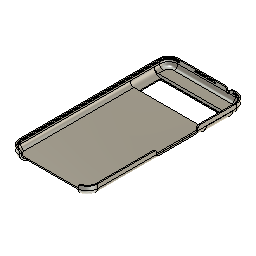
Phone Case (Autodesk Fusion 360 design; units mm, degrees)
Autodesk Fusion 360 part; units mm, degrees
note: some values were not read from the file. Chosen so that the rebuilt part matches the saved one: which bodies a step acts on; which sketch regions a step uses; a direction; which face or edge a step refers to.
sketch "Base Profile" plane through (0, 0, 0) normal (0, 1, 0) x (1, 0, 0)
  line L0 (-39.6, 0) -> (39.6, 0) construction
  line L1 (0, 8.3) -> (-35.6374, 8.3)
  arc A0 (-35.6374, 8.3) -> (-39.6372, 4.2651) centre (-35.6374, 4.3) ccw
  line L2 (0, 9.6) -> (-35.6374, 9.6)
  arc A1 (-35.6374, 9.6) -> (-40.9346, 4.1273) centre (-35.6374, 4.3) ccw
  line L3 (-40.9346, 4.1273) -> (-40.8, 0)
  line L4 (0, 0) -> (0, 9.6)
  line L5 (-39.6372, 4.2651) -> (-39.6, 0)
  line L6 (-40.8, 0) -> (-39.6, 0)
  point P0 (-39.6, 8.3)
  dimension "d2" = 8.3
  dimension "d3" = 4
  dimension "d37" = 90.5
  dimension "d38" = 1.2
  dimension "d39" = 39.6
  dimension "d40" = 4.3
  constraint horizontal L0
  constraint horizontal L1
  constraint coincident P0 L1
  constraint tangent L1 A0
  constraint midpoint L4.start L0
  constraint coincident L4.start origin
  constraint perpendicular L2 L4
  constraint parallel L0 L6
  constraint concentric A0 A1
  constraint tangent L2 A1
  constraint coincident L4 L1.start
  constraint tangent A0 L5
  constraint tangent A1 L3
  measures "d2" distance of L0.start P0
  measures "d3" radius of A0
  measures "d37" angle of L0 L5
  measures "d38" distance of L0.start L3.end
  measures "d39" distance of L4.start L0.start
  measures "d40" distance of L0 A0.centre
sketch "Perimeter" plane through (0, 0, 0) normal (0, 0, 1) x (1, 0, 0)
  line L0 (-30.1, 82.05) -> (30.1, 82.05)
  line L1 (39.6, 72.55) -> (39.6, -72.55)
  line L2 (30.1, -82.05) -> (-30.1, -82.05)
  line L3 (-39.6, -72.55) -> (-39.6, 72.55)
  line L4 (-39.6, 82.05) -> (39.6, -82.05) construction
  line L5 (39.6, 82.05) -> (-39.6, -82.05) construction
  arc A0 (-30.1, 82.05) -> (-39.6, 72.55) centre (-30.1, 72.55) ccw
  line L6 (-30.1, 72.55) -> (30.1, 72.55) construction
  line L7 (30.1, 72.55) -> (30.1, -72.55) construction
  line L8 (30.1, -72.55) -> (-30.1, -72.55) construction
  line L9 (-30.1, -72.55) -> (-30.1, 72.55) construction
  line L10 (30.1, -72.55) -> (-30.1, 72.55) construction
  arc A1 (-39.6, -72.55) -> (-30.1, -82.05) centre (-30.1, -72.55) ccw
  arc A2 (30.1, -82.05) -> (39.6, -72.55) centre (30.1, -72.55) ccw
  arc A3 (39.6, 72.55) -> (30.1, 82.05) centre (30.1, 72.55) ccw
  line L11 (-39.6, -82.05) -> (-39.6, -72.55) construction
  line L12 (-30.1, -82.05) -> (-39.6, -82.05) construction
  line L13 (39.6, -82.05) -> (30.1, -82.05) construction
  line L14 (39.6, -72.55) -> (39.6, -82.05) construction
  line L15 (30.1, 82.05) -> (39.6, 82.05) construction
  line L16 (39.6, 82.05) -> (39.6, 72.55) construction
  line L17 (-39.6, 72.55) -> (-39.6, 82.05) construction
  line L18 (-39.6, 82.05) -> (-30.1, 82.05) construction
  point P0 (39.6, 0)
  dimension "d9" = 164.1
  dimension "d10" = 9.5
  constraint horizontal L0
  constraint perpendicular L0 L1
  constraint parallel L0 L2
  constraint parallel L1 L3
  constraint coincident L4 origin
  constraint coincident L5 origin
  constraint coincident L1 P0
  constraint tangent L3 A0
  constraint tangent L0 A0
  constraint horizontal L6
  constraint vertical L7
  constraint horizontal L8
  constraint vertical L9
  constraint coincident A0.centre L6.start
  constraint midpoint origin L10
  constraint coincident L8.end L9.start
  constraint coincident L7.end L8.start
  constraint coincident L6.end L7.start
  constraint equal A0 A1
  constraint equal A0 A2
  constraint equal A0 A3
  constraint parallel L1 L11
  constraint parallel L0 L12
  constraint parallel L0 L13
  constraint perpendicular L0 L14
  constraint horizontal L15
  constraint perpendicular L0 L16
  constraint parallel L1 L17
  constraint horizontal L18
  measures "d9" distance of L4.start L5.end
  measures "d10" radius of A0
sweep "Sweep1" add profiles "Base Profile" path "Perimeter" along A0 L0 A3 L1 A2 L2 A1 L3 section 1 makes body 1
sketch "Headphone notch" plane through (0, 82.0438, 0.716) normal (0, -0.999962, -0.008727) x (1, 0, 0)
  line L0 (-30.1, 0) -> (-30.1, -4.3)
  arc A0 (21.1007, -4.2633) -> (24.0993, -4.2633) centre (22.6, -4.216) ccw
  line L1 (22.6, -4.216) -> (22.6, 0) construction
  line L2 (-30.1, -0.716) -> (-30.1, -4.9813)
  line L3 (-30.1, -4.9813) -> (30.1, -4.9813)
  line L4 (30.1, -4.9813) -> (30.1, -0.716)
  line L5 (30.1, -0.716) -> (-30.1, -0.716)
  arc A1 (21.05, -2.653) -> (19.051, -0.716) centre (19.051, -2.716) ccw
  line L6 (-30.1, -0.716) -> (30.1, -0.716)
  line L7 (21.1007, -4.2633) -> (21.05, -2.653)
  arc A2 (26.149, -0.716) -> (24.15, -2.653) centre (26.149, -2.716) ccw
  line L8 (24.0993, -4.2633) -> (24.15, -2.653)
  point P0 (39.6372, -4.2651)
  dimension "d17" = 3
  dimension "d43" = 22.6
  dimension "d44" = 2
  dimension "d45" = 3.5
  dimension "d46" = 3.1
  constraint coincident A0.centre L1.start
  constraint coincident L5 A1.end
  constraint tangent L5 A1
  constraint vertical L1
  constraint horizontal A0.start A0.end
  constraint tangent A0 L7
  constraint tangent A1 L7
  constraint symmetric A0.start L1 A0.end
  constraint symmetric L1 A1.start A2.end
  constraint symmetric L1 A1.end A2.start
  constraint symmetric L1 A1 A2
  measures "d17" diameter of A0
  measures "d43" distance of origin L1
  measures "d44" radius of A1
  measures "d45" distance of A0.centre L6
  measures "d46" distance of A1.start A2.end
extrude "Extrude2" cut sketch "Headphone notch" along normal mid plane 10 contours A0 L3 L5 A1 L6 L7 A2 L8 | A0 L3 bodies 1
sketch "Volume control notch" plane through (39.597, 0, 0.3456) normal (-0.999962, 0, -0.008727) x (0, -1, 0)
  line L0 (-28.6516, -7.3456) -> (7.6516, -7.3456)
  line L1 (-10.5, -7.3456) -> (-10.5, -0.3456) construction
  arc A0 (-32.15, -3.9506) -> (-28.6516, -7.3456) centre (-28.6516, -3.8456) ccw
  line L2 (-32.15, -3.9506) -> (-32.2, -2.2855)
  arc A1 (-32.2, -2.2855) -> (-34.1991, -0.3456) centre (-34.1991, -2.3456) ccw
  arc A2 (7.6516, -7.3456) -> (11.15, -3.9506) centre (7.6516, -3.8456) ccw
  line L3 (11.15, -3.9506) -> (11.2, -2.2855)
  arc A3 (13.1991, -0.3456) -> (11.2, -2.2855) centre (13.1991, -2.3456) ccw
  line L4 (-72.55, -0.3456) -> (-72.55, -4.6108)
  line L5 (-72.55, -4.6108) -> (72.55, -4.6108)
  line L6 (72.55, -4.6108) -> (72.55, -0.3456)
  line L7 (72.55, -0.3456) -> (-72.55, -0.3456)
  dimension "d25" = 7
  dimension "d26" = 2
  dimension "d27" = 3.5
  dimension "d29" = 43.4
  dimension "d30" = 43.3
  dimension "d47" = 10.5
  constraint coincident L0 L1.start
  constraint midpoint L0 L1.start
  constraint tangent L0 A0
  constraint tangent A0 L2
  constraint tangent L2 A1
  constraint symmetric L0.start L1 L0.end
  constraint symmetric L1 A0.start A2.end
  constraint symmetric L1 A0 A2
  constraint symmetric L1 L2.end L3.end
  constraint symmetric L1 A1.end A3.start
  constraint symmetric L1 A1 A3
  constraint coincident A1.end L7
  constraint tangent A1 L7
  constraint horizontal L0
  constraint vertical L1
  constraint coincident L1.end L7
  measures "d25" distance of L1.start L1.end
  measures "d26" radius of A1
  measures "d27" radius of A0
  measures "d29" distance of L2.end L3.end
  measures "d30" distance of A0.start A2.end
  measures "d47" distance of origin L1
extrude "Extrude3" cut sketch "Volume control notch" along normal mid plane 10 contours L0 A0 A2 L5 | A0 L2 A1 A2 L3 A3 L5 L7 bodies 1
sketch "Charger notch" plane through (0, 0, -9.6) normal (0, 0, -1) x (1, 0, 0)
  arc A0 (-35.6374, -72.55) -> (-30.1, -78.0874) centre (-30.1, -72.55) ccw
  line L0 (-30.1, -78.0874) -> (30.1, -78.0874)
  arc A1 (30.1, -78.0874) -> (35.6374, -72.55) centre (30.1, -72.55) ccw
  line L1 (35.6374, -72.55) -> (35.6374, 72.55)
  arc A2 (35.6374, 72.55) -> (30.1, 78.0874) centre (30.1, 72.55) ccw
  line L2 (30.1, 78.0874) -> (-30.1, 78.0874)
  arc A3 (-30.1, 78.0874) -> (-35.6374, 72.55) centre (-30.1, 72.55) ccw
  line L3 (-35.6374, 72.55) -> (-35.6374, -72.55)
  line L4 (30.1, 82.05) -> (-30.1, 82.05) construction
  line L5 (30.1, 83.25) -> (-30.1, 83.25) construction
  line L6 (30.1, 83.3846) -> (-30.1, 83.3846)
  line L7 (-25.2845, 77.9846) -> (27.2845, 77.9846)
  line L8 (-29.6, 83.3846) -> (31.6, 83.3846)
  line L9 (1, 83.3846) -> (1, 77.9846) construction
  arc A4 (-27.0092, 78.9719) -> (-25.2845, 77.9846) centre (-25.2845, 79.9846) ccw
  line L10 (-27.0092, 78.9719) -> (-29.6, 83.3846)
  line L11 (29.0092, 78.9719) -> (31.6, 83.3846)
  arc A5 (27.2845, 77.9846) -> (29.0092, 78.9719) centre (27.2845, 79.9846) ccw
  line L12 (31.6, 83.3846) -> (31.6, 86.3846)
  line L13 (-29.6, 83.3846) -> (-29.6, 86.3846)
  line L14 (-29.6, 86.3846) -> (31.6, 86.3846)
  dimension "d48" = 52.569
  dimension "d49" = 61.2
  dimension "d50" = 2
  dimension "d51" = 5.4
  dimension "d52" = 1
  dimension "d55" = 3
  constraint parallel L4 L7
  constraint horizontal L8
  constraint midpoint L8 L9.start
  constraint midpoint L7 L9.end
  constraint vertical L9
  constraint tangent L7 A4
  constraint tangent A4 L10
  constraint collinear L6 L8
  constraint symmetric L7.start L9 L7.end
  constraint symmetric L8.start L9 L8.end
  constraint symmetric L9 A4.start L11.start
  constraint symmetric L9 A4 A5
  constraint perpendicular L8 L12
  constraint perpendicular L8 L13
  constraint horizontal L14
  measures "d48" distance of L7.start L7.end
  measures "d49" distance of L8.start L8.end
  measures "d50" radius of A4
  measures "d51" distance of L7 L8
  measures "d52" distance of origin L9
  measures "d55" distance of L8.end L12.end
extrude "Extrude4" cut sketch "Charger notch" against normal blind 11.927 contours L2 L6 L8 A4 L10 L11 A5 | L6 L8 L12 L13 L14 bodies 1
fillet "Fillet2" radius 2 2 edges at (31.1353, -82.5931, 0) (-29.1687, -82.65, 0) on bodies 1
sketch "Retaining Ring profile for sweep" plane through (0, 0, 0) normal (0, 1, 0) x (1, 0, 0)
  line L0 (-39.6372, 4.2651) -> (-39.6, 0)
  line L1 (-39.6175, 2) -> (-38.6087, 1.4293)
  line L2 (-38.6087, 1.4293) -> (-38.6087, 1.0087)
  line L3 (-38.6087, 1.0087) -> (-39.6087, 1)
  dimension "d60" = 60
  dimension "d62" = 1
  dimension "d63" = 1
  dimension "d64" = 1
  constraint coincident L0 L1.start
  constraint vertical L2
  constraint coincident L0 L3.end
  constraint perpendicular L0 L3
  measures "d60" angle of L0 L1
  measures "d62" vertical distance of L1.start L3.end
  measures "d63" vertical distance of L0.end L3.end
  measures "d64" horizontal distance of L2.end L3.end
sweep "Sweep2" add profiles "Retaining Ring profile for sweep" path "Perimeter" along A0 L0 A3 L1 A2 L2 A1 L3 section 1 separate body makes body 2
sketch "Retaining Ring cutouts" plane through (0, 0, 0) normal (0, 0, 1) x (1, 0, 0)
  line L0 (-28.3042, 76.8842) -> (-11.4621, 76.8842)
  line L1 (-11.4621, 76.8842) -> (-11.4621, 87.5508)
  line L2 (-11.4621, 87.5508) -> (-28.3042, 87.5508)
  line L3 (-28.3042, 87.5508) -> (-28.3042, 76.8842)
  line L4 (9.7778, 73.0492) -> (28.2586, 73.0492)
  line L5 (28.2586, 73.0492) -> (28.2586, 87.5508)
  line L6 (28.2586, 87.5508) -> (9.7778, 87.5508)
  line L7 (9.7778, 87.5508) -> (9.7778, 73.0492)
  line L8 (34.3544, -16.9326) -> (47.9088, -16.9326)
  line L9 (47.9088, -16.9326) -> (47.9088, 41.7139)
  line L10 (47.9088, 41.7139) -> (34.3544, 41.7139)
  line L11 (34.3544, 41.7139) -> (34.3544, -16.9326)
  line L12 (-32.3646, -87.8519) -> (33.749, -87.8519)
  line L13 (33.749, -87.8519) -> (33.749, -78.2722)
  line L14 (33.749, -78.2722) -> (-32.3646, -78.2722)
  line L15 (-32.3646, -78.2722) -> (-32.3646, -87.8519)
  constraint horizontal L0
  constraint vertical L1
  constraint horizontal L2
  constraint vertical L3
  constraint horizontal L4
  constraint vertical L5
  constraint horizontal L6
  constraint vertical L7
  constraint horizontal L8
  constraint vertical L9
  constraint horizontal L10
  constraint vertical L11
  constraint horizontal L12
  constraint vertical L13
  constraint horizontal L14
  constraint vertical L15
extrude "Extrude5" cut sketch "Retaining Ring cutouts" against normal blind 10 bodies 2 makes body 3 at (-4.3822, 81.395, -1.6195) makes body 4 at (38.945, 62.2713, -1.6195) makes body 5 at (-38.945, 24.1833, -1.6195)
combine "Combine1" operation add target body 1 tool bodies 2 3 4 5
ref_plane "WorkPlane1" through (0, 40.9, 0) normal (0, 1, 0) x (0, 0, 1)
sketch "Camera Hump" plane through (0, 40.9, 0) normal (0, 1, 0) x (1, 0, 0)
  line L0 (-30.1, 9.6) -> (-35.6374, 9.6)
  line L1 (-30.1, 9.6) -> (30.1, 9.6)
  line L2 (35.6374, 9.6) -> (30.1, 9.6)
  line L3 (35.6374, 9.6) -> (30.1, 9.6)
  line L4 (30.1, 9.6) -> (27.9175, 9.6)
  line L5 (27.9175, 9.6) -> (-25.9175, 9.6)
  line L6 (-25.9175, 9.6) -> (-30.1, 9.6)
  line L7 (-30.1, 9.6) -> (-35.6374, 9.6)
  spline S0 degree 3 poles (40.201, 6.995) (40.201, 6.995) (40.2595, 6.9015) (40.4476, 6.5348) (40.5721, 6.2617) (40.7754, 5.6397) (40.8693, 5.25) (40.9338, 4.5974) (40.9422, 4.3628) (40.9346, 4.1273) knots 0 0 0 0 0.136028 0.136028 0.272056 0.272056 0.404552 0.404552 0.473854 0.473854 0.473854 0.473854
  arc A0 (40.9346, 4.1273) -> (35.6374, 9.6) centre (35.6374, 4.3) ccw
  arc A1 (40.9346, 4.1273) -> (35.6374, 9.6) centre (35.6374, 4.3) ccw
  spline S1 degree 3 poles (40.9346, 4.1273) (40.9422, 4.3628) (40.9338, 4.5974) (40.8693, 5.25) (40.7754, 5.6397) (40.5721, 6.2617) (40.4476, 6.5348) (40.2595, 6.9015) (40.201, 6.995) (40.201, 6.995) knots -0.473854 -0.473854 -0.473854 -0.473854 -0.404552 -0.404552 -0.272056 -0.272056 -0.136028 -0.136028 0 0 0 0
  arc A2 (-35.6374, 9.6) -> (-40.9346, 4.1273) centre (-35.6374, 4.3) ccw
  arc A3 (-35.6374, 9.6) -> (-40.9346, 4.1273) centre (-35.6374, 4.3) ccw
  line L8 (-30.1, 8.3) -> (-35.6374, 8.3)
  line L9 (-30.1, 8.3) -> (-25.9175, 8.3)
  line L10 (-25.9175, 8.3) -> (27.9175, 8.3)
  line L11 (27.9175, 8.3) -> (30.1, 8.3)
  line L12 (35.6374, 8.3) -> (30.1, 8.3)
  line L13 (35.6374, 8.3) -> (30.1, 8.3)
  line L14 (30.1, 8.3) -> (-30.1, 8.3)
  line L15 (-30.1, 8.3) -> (-35.6374, 8.3)
  arc A4 (-35.6374, 8.3) -> (-39.6372, 4.2651) centre (-35.6374, 4.3) ccw
  arc A5 (-35.6374, 8.3) -> (-39.6372, 4.2651) centre (-35.6374, 4.3) ccw
  spline S2 degree 3 poles (39.6372, 4.2651) (39.6404, 4.6245) (39.5922, 4.9872) (39.4158, 5.6618) (39.283, 5.968) (39.024, 6.4461) (38.8756, 6.655) (38.6508, 6.9366) (38.5803, 7.0091) (38.5802, 7.0092) knots 0.67617 0.67617 0.67617 0.67617 0.785853 0.785853 0.904084 0.904084 1.023831 1.023831 1.143577 1.143577 1.143577 1.143577
  spline S3 degree 3 poles (38.5802, 7.0092) (38.5803, 7.0091) (38.6508, 6.9366) (38.8756, 6.655) (39.024, 6.4461) (39.283, 5.968) (39.4158, 5.6618) (39.5922, 4.9872) (39.6404, 4.6245) (39.6372, 4.2651) knots 1.143577 1.143577 1.143577 1.143577 1.263323 1.263323 1.38307 1.38307 1.501301 1.501301 1.610984 1.610984 1.610984 1.610984
  arc A6 (39.6372, 4.2651) -> (35.6374, 8.3) centre (35.6374, 4.3) ccw
  arc A7 (39.6372, 4.2651) -> (35.6374, 8.3) centre (35.6374, 4.3) ccw
  line L16 (0, 8.3) -> (0, 12.3) construction
  line L17 (-32.9364, 12.3) -> (32.9364, 12.3)
  arc A8 (-32.9364, 12.3) -> (-40.9346, 4.1273) centre (-32.9364, 4.3) ccw
  arc A9 (40.9346, 4.1273) -> (32.9364, 12.3) centre (32.9364, 4.3) ccw
  dimension "d79" = 4
  constraint midpoint L14 L16.start
  constraint perpendicular L5 L16
  constraint horizontal L17
  constraint midpoint L16.end L17
  constraint coincident A2 A3.end
  constraint tangent L17 A8
  constraint coincident A2.end A3.end
  constraint horizontal A2.centre A8.centre
  constraint symmetric L16 L17.start L17.end
  constraint symmetric L16 A2.end S0.end
  constraint symmetric L16 A8 A9
  measures "d79" distance of L16.start L16.end
extrude "Extrude7" add sketch "Camera Hump" along normal blind 27.3 bodies 1
sketch "Camera Hump Hole" plane through (0, 0, -12.3) normal (0, 0, -1) x (1, 0, 0)
  line L0 (32.9364, -40.9) -> (-32.9364, -40.9)
  line L1 (-32.9364, -40.9) -> (-32.9364, -68.2)
  line L2 (-32.9364, -68.2) -> (32.9364, -68.2)
  line L3 (32.9364, -68.2) -> (32.9364, -40.9)
  line L4 (36.25, -66.7) -> (-34.25, -66.7)
  line L5 (-34.25, -66.7) -> (-34.25, -42.4)
  line L6 (-34.25, -42.4) -> (36.25, -42.4)
  line L7 (36.25, -42.4) -> (36.25, -66.7)
  line L8 (-34.25, -54.55) -> (-32.9364, -54.55) construction
  point P0 (1, -42.4)
  dimension "d82" = 1
  dimension "d83" = 24.3
  dimension "d84" = 70.5
  constraint horizontal L4
  constraint vertical L5
  constraint horizontal L6
  constraint vertical L7
  constraint midpoint L5 L8.start
  constraint midpoint L1 L8.end
  constraint horizontal L8
  constraint midpoint L6 P0
  measures "d82" horizontal distance of origin P0
  measures "d83" distance of L4.start L6.end
  measures "d84" distance of L5.end L6.end
extrude "Extrude8" cut sketch "Camera Hump Hole" against normal through all contours L1 L3 L4 L6 bodies 1
fillet "Fillet3" radius 3 4 edges at (32.9364, 66.7, -10.3) (32.9364, 42.4, -10.3) (-32.9364, 42.4, -10.3) (-32.9364, 66.7, -10.3) on bodies 1
ref_plane "WorkPlane2" through (0, 54.55, -10.3) normal (0, -1, 0) x (1, 0, 0)
sketch "Camera Hump Internal Cutout" plane through (0, 54.55, 0) normal (0, -1, 0) x (1, 0, 0)
  line L0 (-29.9364, -8.3) -> (-29.9364, -12.3) construction
  line L1 (-29.9364, -12.3) -> (29.9364, -12.3)
  line L2 (29.9364, -12.3) -> (29.9364, -8.3) construction
  line L3 (29.9364, -8.3) -> (-29.9364, -8.3)
  line L4 (-29.9364, -8.3) -> (29.9364, -8.3)
  line L5 (32.9364, -8.3) -> (29.9364, -8.3)
  line L6 (32.9364, -8.3) -> (29.9364, -8.3)
  line L7 (29.9364, -8.3) -> (-29.9364, -8.3)
  line L8 (-29.9364, -8.3) -> (-32.9364, -8.3)
  line L9 (-29.9364, -8.3) -> (-32.9364, -8.3)
  line L10 (-35.6374, -8.3) -> (-30.1, -8.3)
  line L11 (-30.1, -8.3) -> (-25.9175, -8.3)
  line L12 (-25.9175, -8.3) -> (27.9175, -8.3)
  line L13 (27.9175, -8.3) -> (30.1, -8.3)
  line L14 (30.1, -8.3) -> (35.6374, -8.3)
  line L15 (30.1, -8.3) -> (35.6374, -8.3)
  line L16 (30.1, -8.3) -> (-30.1, -8.3)
  line L17 (-35.6374, -8.3) -> (-30.1, -8.3)
  arc A0 (32.9364, -12.3) -> (40.9346, -4.4727) centre (32.9364, -4.3) ccw
  arc A1 (32.9364, -12.3) -> (40.9346, -4.4727) centre (32.9364, -4.3) ccw
  arc A2 (-40.9346, -4.4727) -> (-32.9364, -12.3) centre (-32.9364, -4.3) ccw
  arc A3 (-40.9346, -4.4727) -> (-32.9364, -12.3) centre (-32.9364, -4.3) ccw
  line L18 (29.9364, -12.3) -> (-29.9364, -12.3)
  line L19 (32.9364, -12.3) -> (32.9364, -8.3)
  line L20 (32.9364, -8.3) -> (32.9364, -12.3) construction
  arc A4 (-39.6372, -4.2651) -> (-35.6374, -8.3) centre (-35.6374, -4.3) ccw
  arc A5 (-39.6372, -4.2651) -> (-35.6374, -8.3) centre (-35.6374, -4.3) ccw
  spline S0 degree 3 poles (39.6372, -4.2651) (39.6404, -4.6245) (39.5922, -4.9872) (39.4158, -5.6618) (39.283, -5.968) (39.024, -6.4461) (38.8756, -6.655) (38.6508, -6.9366) (38.5803, -7.0091) (38.5802, -7.0092) knots 0.67617 0.67617 0.67617 0.67617 0.785853 0.785853 0.904084 0.904084 1.023831 1.023831 1.143577 1.143577 1.143577 1.143577
  spline S1 degree 3 poles (38.5802, -7.0092) (38.5803, -7.0091) (38.6508, -6.9366) (38.8756, -6.655) (39.024, -6.4461) (39.283, -5.968) (39.4158, -5.6618) (39.5922, -4.9872) (39.6404, -4.6245) (39.6372, -4.2651) knots 1.143577 1.143577 1.143577 1.143577 1.263323 1.263323 1.38307 1.38307 1.501301 1.501301 1.610984 1.610984 1.610984 1.610984
  arc A6 (35.6374, -8.3) -> (39.6372, -4.2651) centre (35.6374, -4.3) ccw
  arc A7 (35.6374, -8.3) -> (39.6372, -4.2651) centre (35.6374, -4.3) ccw
  line L21 (32.9364, -11.3) -> (-32.9364, -11.3)
  line L22 (0, 0) -> (0, -11.3) construction
  arc A8 (-39.6372, -4.2651) -> (-32.9364, -11.3) centre (-32.9364, -4.5913) ccw
  arc A9 (32.9364, -11.3) -> (39.6372, -4.2651) centre (32.9364, -4.5913) ccw
  dimension "d89" = 1
  constraint horizontal L21
  constraint coincident L22.start origin
  constraint perpendicular L12 L22
  constraint midpoint L21 L22.end
  constraint coincident A4.start A5.start
  constraint tangent L21 A8
  constraint vertical A2.centre A8.centre
  constraint symmetric L21.end L22 L21.start
  constraint symmetric L22 A4.start S0.start
  constraint symmetric L22 A8 A9
  measures "d89" distance of L1 L21
extrude "Extrude9" cut sketch "Camera Hump Internal Cutout" along normal mid plane 25.2 bodies 1
equation "d9 = 40.4 mm + 148.3 mm - 24.6 mm"
equation "d78 = 42.5 mm - 1.6 mm"
named bodies: "Phone case", "Retaining Ring", "Retaining Ring (1)", "Retaining Ring (2)", "Retaining Ring (3)"
